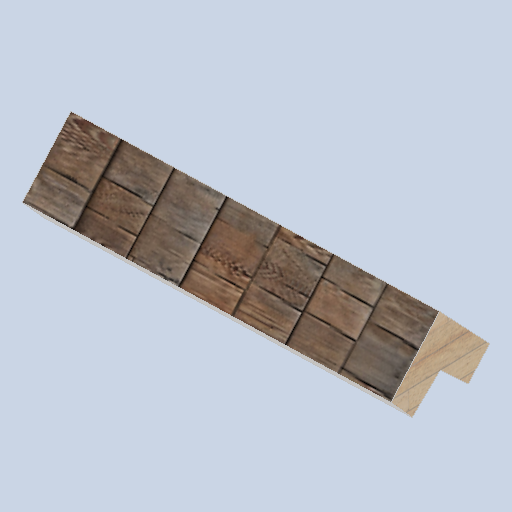
# Autodesk Inventor part: panel_block_02
Saved by Autodesk Inventor 2024.2 (Build 282272000, 272)
## iProperties
Created: 2024-05-21
Part Number: panel_block_02
Material: Wood (Maple)
Document SubType Name: Modeling
Designer: LOSTER_1
Density: 0.67 g/cm^3
Appearance: Natural Maple - Glossy Dark Tint
Author: LOSTER_1
Autodesk Inventor part; units mm, degrees
sketch "Sketch1" plane through (0, 0, 0) normal (0, 0, 1) x (1, 0, 0)
  line L0 (2948.6488, 634.5525) -> (2841.4489, 559.4904)
  line L1 (2841.4489, 559.4904) -> (2956.2003, 395.6085)
  line L2 (2956.2003, 395.6085) -> (3063.4001, 470.6706)
  line L3 (1051.1773, 2444.1167) -> (976.8907, 2338.0244)
  line L4 (976.8907, 2338.0244) -> (1140.7211, 2223.3091)
  line L5 (1140.7211, 2223.3091) -> (1215.0077, 2329.4014)
  line L6 (-383.8501, 3232.1868) -> (-383.8501, 3052.6308)
  arc A0 (4065.9398, -2152.4924) -> (-383.8501, 3052.6308) centre (-4485.4868, -4958.3977) ccw
  arc A1 (1051.1773, 2444.1167) -> (-383.8501, 3232.1868) centre (-3980.604, -5017.8654) ccw
  arc A2 (2948.6488, 634.5525) -> (1215.0077, 2329.4014) centre (-4152.392, -4894.9339) ccw
  arc A3 (4300.883, -1939.8955) -> (3063.4001, 470.6706) centre (-4233.2291, -4798.0297) ccw
  arc A4 (4065.9398, -2152.4924) -> (4300.883, -1939.8955) centre (3657.2708, -1464.7499) ccw
  point P0 (0, 0)
  point P1 (4065.924, -2152.4924)
  point P2 (4065.924, -2152.4924)
  dimension "d8" = 9000
  dimension "d9" = 9000
  dimension "d10" = 9000
  dimension "d11" = 9000
  dimension "d12" = 800
  constraints: 14 end point, 10 point on circle, 5 centre point, 4 perpendicular, 1 coincident, 1 vertical
  measures "d8" radius of A0
  measures "d9" radius of A1
  measures "d10" radius of A2
  measures "d11" radius of A3
  measures "d12" radius of A4
ref_plane "Work Plane2" through (0, 0, -7900) normal (0, 0, 1) x (1, 0, 0)
ref_plane "Work Plane1" through (0, 0, 0) normal (0, 0, 1) x (1, 0, 0)
sketch "Sketch2" plane through (0, 0, -7900) normal (0, 0, 1) x (1, 0, 0)
  arc A0 (895.257, 3171.2695) -> (-383.8658, 4018.7524) centre (-4697.1096, -3880.3569) ccw projected
  line L0 (-383.8658, 4018.7524) -> (-383.8658, 3839.1061) projected
  arc A1 (4065.924, -2152.4924) -> (-383.8658, 3839.1061) centre (-4733.9746, -4039.7614) ccw projected
  line L1 (895.257, 3171.2695) -> (830.4728, 3059.0601) projected
  line L2 (830.4728, 3059.0601) -> (1003.6891, 2959.0536) projected
  line L3 (1068.4733, 3071.2631) -> (1003.6891, 2959.0536) projected
  arc A2 (2750.1419, 1279.62) -> (1068.4733, 3071.2631) centre (-4591.4319, -3926.2703) ccw projected
  line L4 (2750.1419, 1279.62) -> (2643.8882, 1205.2246) projected
  line L5 (2643.8882, 1205.2246) -> (2759.146, 1041.7698) projected
  line L6 (2865.5448, 1116.2711) -> (2759.146, 1041.7698) projected
  arc A3 (4310.9102, -1926.005) -> (2865.5448, 1116.2711) centre (-4397.3898, -4198.7812) ccw projected
  arc A4 (4065.924, -2152.4924) -> (4310.9102, -1926.005) centre (3657.2831, -1464.7333) ccw
  point P0 (0, 0)
  dimension "d7" = 800
  constraints: 2 point on circle, 1 centre point
  measures "d7" radius of A4
loft "Loft1" add profiles "Sketch1", "Sketch2"
ref_plane "Work Plane3" through (2500, 0, 0) normal (1, 0, 0) x (0, 1, 0)
sketch "Sketch3" plane through (2500, 0, 0) normal (1, 0, 0) x (0, 1, 0)
  line L0 (2569.5835, -3718.0946) -> (1551.2045, -2616.5476)
  line L1 (1551.2045, -2616.5476) -> (1738.7871, -4630.7013)
  line L2 (1738.7871, -4630.7013) -> (2569.5835, -3718.0946)
  line L3 (4228.9662, 279.606) -> (-2269.9695, 279.606)
  line L4 (-2269.9695, 279.606) -> (-2269.9695, -8192.2559)
  line L5 (-2269.9695, -8192.2559) -> (4228.9662, -8192.2559)
  line L6 (4228.9662, -8192.2559) -> (4228.9662, 279.606)
  point P0 (0, 0)
  constraints: 14 end point, 2 parallel, 1 horizontal, 1 perpendicular
extrude "Extrusion1" cut sketch "Sketch3" along normal through all both and the other way through all
ref_plane "Work Plane4" through (1945.737, 1551.2045, -2616.5476) normal (0, -0.9956912, -0.0927309) x (1, 0, 0)
sketch "Sketch5" plane through (1945.737, 1551.2045, -2616.5476) normal (0, -0.9956912, -0.0927309) x (1, 0, 0)
  line L0 (347.8734, 0) -> (290.3896, -2022.8698)
  point P0 (-1945.737, 2749.1181)
  constraints: 2 end point
ref_plane "Work Plane5" through (2293.6104, 1551.2045, -2616.5476) normal (-0.6425282, -0.7644369, -0.052856) x (-0.0284055, 0.0926935, -0.9952894)
sketch "Sketch6" plane through (2293.6104, 1551.2045, -2616.5476) normal (-0.6425282, -0.7644369, -0.052856) x (-0.0284055, 0.0926935, -0.9952894)
  line L0 (-1061.9028, -2252.9112) -> (2197.0944, -2252.9112)
  line L1 (2197.0944, -2252.9112) -> (2197.0944, 343.7273)
  line L2 (2197.0944, 343.7273) -> (-1061.9028, 343.7273)
  line L3 (-1061.9028, 343.7273) -> (-1061.9028, -2252.9112)
  point P0 (-2682.8576, -979.2829)
  constraints: 8 end point, 2 parallel, 1 horizontal, 1 perpendicular
extrude "Extrusion2" cut sketch "Sketch6" against normal through all
ref_plane "Work Plane6" through (2293.6104, 1551.2045, -2616.5476) normal (-0.9995965, -0.0026341, 0.0282831) x (-0.0284055, 0.0926935, -0.9952894)
sketch "Sketch7" plane through (2293.6104, 1551.2045, -2616.5476) normal (-0.6425282, -0.7644369, -0.052856) x (-0.0284055, 0.0926935, -0.9952894)
  line L0 (0, 0) -> (1222.5973, -1418.5767) projected
  line L1 (1222.5973, -1418.5767) -> (2023.6864, 0) projected
  point P0 (-2682.8576, -979.2829)
  constraints: 1 horizontal alignment
sketch "Sketch8" plane through (2293.6104, 1551.2045, -2616.5476) normal (-0.9995965, -0.0026341, 0.0282831) x (-0.0284055, 0.0926935, -0.9952894)
  line L0 (0, 0) -> (1222.5973, -911.8435) projected
  spline S0 degree 4 poles (2023.6864, 0) (1891.4174, -0.0605) (1759.1485, -0.1112) (1626.8795, -0.1518) (1361.543, -0.2126) (1228.4756, -0.2325) (1095.4081, -0.2417) (831.8573, -0.2379) (701.374, -0.2253) (570.8907, -0.2017) (330.3055, -0.1374) (220.2037, -0.0999) (110.1018, -0.0542) (0, 0) knots 0 0 0 0 0 0.261442 0.261442 0.261442 0.524462 0.524462 0.524462 0.782374 0.782374 0.782374 1 1 1 1 1 projected
  line L1 (1222.5973, -911.8435) -> (2023.6864, 0) projected
  point P0 (-2682.8576, 1301.8858)
  constraints: 1 horizontal alignment
sketch "Sketch9" plane through (2293.6104, 1551.2045, -2616.5476) normal (-0.9995965, -0.0026341, 0.0282831) x (-0.0284055, 0.0926935, -0.9952894)
  line L0 (1222.5973, -911.8435) -> (0, 0) projected
  line L1 (2023.6864, 0) -> (1222.5973, -911.8435) projected
  spline S0 degree 4 poles (0, 0) (253.1862, 0) (506.3724, 0) (759.5586, 0) (1265.4802, 0) (1518.2156, 0) (1770.951, 0) (2023.6864, 0) knots 0 0 0 0 0 0.500446 0.500446 0.500446 1 1 1 1 1 projected
  point P0 (-2682.8576, 1301.8858)
  constraints: 1 horizontal alignment
extrude "Extrusion3" add sketch "Sketch9" against normal blind 1
sketch "Sketch10" plane through (2294.61, 1551.2071, -2616.5759) normal (0.9995965, 0.0026341, -0.0282831) x (-0.0284055, 0.0926935, -0.9952894)
  line L0 (1222.5973, 911.8435) -> (2011.6459, 13.7052) projected
  line L1 (1222.5973, 911.8435) -> (1126.4049, 840.1008)
  line L2 (0, 0) -> (1222.5973, 911.8435) projected
  line L3 (1222.5973, 911.8435) -> (1301.7983, 821.6925)
  line L4 (1301.7983, 821.6925) -> (1376.9241, 887.6934)
  line L5 (1376.9241, 887.6934) -> (1235.027, 1068.2138)
  line L6 (1126.4049, 840.1008) -> (1066.6193, 920.2612)
  line L7 (1066.6193, 920.2612) -> (1235.027, 1068.2138)
  point P0 (-2682.8576, -1301.8858)
  dimension "d31" = 120
  dimension "d32" = 120
  dimension "d33" = 100
  dimension "d34" = 100
  constraints: 12 end point, 2 perpendicular, 2 point on line
  measures "d31" distance of L0.start L1.end
  measures "d32" distance of L0.start L3.end
  measures "d33" distance of L3.end L4.end
  measures "d34" distance of L1.end L6.end
extrude "Extrusion5" add sketch "Sketch10" against normal blind 1100
sketch "Sketch16" plane through (2294.61, 1551.2071, -2616.5759) normal (0.9995965, 0.0026341, -0.0282831) x (-0.0284055, 0.0926935, -0.9952894)
  line L0 (0, 0) -> (1126.4049, 840.1008) projected
  line L1 (1020.1978, 760.8889) -> (1222.5973, 911.8435)
  line L2 (0, 0) -> (-179.2361, -133.6787)
  line L3 (-179.2361, -133.6787) -> (2478.6059, -144.4888)
  line L4 (2478.6059, -144.4888) -> (2023.6864, 0)
  line L5 (1305.5559, 824.9938) -> (1226.6196, 914.8434)
  line L6 (1222.5973, 911.8435) -> (1226.6196, 914.8434)
  point P0 (-2682.8576, -1301.8858)
  constraints: 12 end point, 1 point on line, 1 other
extrude "Extrusion6" cut sketch "Sketch8" along normal blind 2000
sketch "Sketch17" plane through (2256.6322, 2490.0248, -3836.0174) normal (0.0213399, -0.7268016, 0.6865159) x (0.9995965, 0.0026341, -0.0282831)
  line L0 (0, 0) -> (-979.255, 0) projected
  line L1 (-1518.239, 0) -> (548.3239, 0)
  line L2 (548.3239, 0) -> (548.3239, -1298.4887)
  line L3 (548.3239, -1298.4887) -> (-1518.239, -1298.4887)
  line L4 (-1518.239, -1298.4887) -> (-1518.239, 0)
  point P0 (-2370.775, 1034.5522)
  point P1 (-1213.4732, 0)
  point P2 (-1999, 0)
  constraints: 8 end point, 2 parallel, 1 horizontal, 1 perpendicular, 1 point on line
extrude "Extrusion7" cut sketch "Sketch17" along normal mid plane 5000
sketch "Sketch18" plane through (2294.61, 1551.2071, -2616.5759) normal (0.9995965, 0.0026341, -0.0282831) x (-0.0284055, 0.0926935, -0.9952894)
  line L0 (1126.4049, 840.1008) -> (1222.5973, 911.8435) projected
  line L1 (1301.7983, 821.6925) -> (366.6688, 0.1458) projected
  spline S0 degree 4 poles (366.6688, 0.1458) (275.0016, 0.1179) (183.3344, 0.0844) (91.6672, 0.0451) (0, 0) knots 0 0 0 0 0 1 1 1 1 1 projected
  line L2 (0, 0) -> (1126.4049, 840.1008) projected
  line L3 (1126.4049, 840.1008) -> (1222.5973, 911.8435) projected
  line L4 (1222.5973, 911.8435) -> (1301.7983, 821.6925) projected
  point P0 (-2682.8576, -1301.8858)
  point P1 (1126.4049, 840.1008)
  constraints: 1 other
extrude "Extrusion8" cut sketch "Sketch18" along normal mid plane 5000
sketch "Sketch19" plane through (1945.737, 1551.2045, -2616.5476) normal (0, -0.9956912, -0.0927309) x (1, 0, 0)
  line L0 (407.6375, 227.4777) -> (-99.9449, 227.4777)
  line L1 (-99.9449, 227.4777) -> (-99.9449, -459.2513)
  line L2 (-99.9449, -459.2513) -> (407.6375, -459.2513)
  line L3 (407.6375, -459.2513) -> (407.6375, 227.4777)
  point P0 (-1945.737, 2749.1181)
  constraints: 8 end point, 2 parallel, 1 horizontal, 1 perpendicular
extrude "Extrusion9" cut sketch "Sketch19" along normal mid plane 100
sketch "Sketch20" plane through (929.9316, 2569.5835, -3718.0946) normal (0, 0.7394745, -0.6731846) x (1, 0, 0)
  line L0 (3.9942, -0.4392) -> (230.3898, -0.0226) projected
  line L1 (-207.8079, -0.0226) -> (-207.8079, 338.0495)
  line L2 (-207.8079, 338.0495) -> (230.3898, 338.0495)
  line L3 (230.3898, 338.0495) -> (230.3898, -0.0226)
  line L4 (-207.8079, -0.0226) -> (-207.8079, -237.6599)
  line L5 (-207.8079, -237.6599) -> (230.3898, -237.6599)
  line L6 (230.3898, -237.6599) -> (230.3898, 129.1543)
  point P0 (-929.9316, -1019.6322)
  constraints: 12 end point, 1 horizontal, 1 parallel, 1 point on line, 1 vertical
extrude "Extrusion10" cut sketch "Sketch20" against normal blind 1100
body "Solid1"
